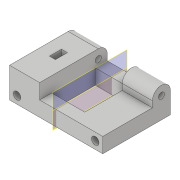
# Autodesk Inventor part: Carriage
Saved by Autodesk Inventor 2019 (Build 230136000, 136)
## iProperties
Created: 2019-01-26
Part Number: Carriage
Material: Generic
Document SubType Name: Modeling
Designer: Jared
Density: 1 g/cm^3
Appearance: Default
Author: Jared
Autodesk Inventor part; units mm, degrees
ref_plane "YZ Plane" through (0, 0, 0) normal (1, 0, 0) x (0, 1, 0)
ref_plane "XZ Plane" through (0, 0, 0) normal (0, 1, 0) x (-1, 0, 0)
ref_plane "XY Plane" through (0, 0, 0) normal (0, 0, 1) x (1, 0, 0)
sketch "Sketch1" plane through (0, 0, 0) normal (0, 1, 0) x (-1, 0, 0)
  line L0 (0, 0) -> (0, -22.5)
  line L1 (0, -22.5) -> (31, -22.5)
  line L2 (31, -22.5) -> (31, 0)
  line L3 (31, 0) -> (0, 0)
  dimension "d0" = 22.5
  dimension "d1" = 31
  constraints: 8 end point, 3 perpendicular, 1 vertical
  measures "d0" distance of L0.start L0.end
  measures "d1" distance of L0.end L1.end
extrude "Extrusion1" add sketch "Sketch1" along normal blind 5
sketch "Sketch2" plane through (-31, 0, 0) normal (0, 0, 1) x (1, 0, 0)
  line L0 (0, 0) -> (31, 0) projected
  line L1 (31, 0) -> (31, 5) projected
  line L2 (0, 5) -> (31, 5) projected
  line L3 (0, 0) -> (0, 5) projected
  line L4 (0, 0) -> (0, 5) projected
  line L5 (0, 2.5) -> (2.5, 2.5)
  circle A0 centre (2.5, 2.5) radius 1.25
  dimension "d4" = 2.5
  dimension "d5" = 2.5
  constraints: 2 end point, 1 centre point, 1 coincident, 1 horizontal, 1 midpoint
  measures "d4" distance of L5.start L5.end
  measures "d5" diameter of A0
extrude "Extrusion2" cut sketch "Sketch2" against normal up to next contours A0
ref_plane "Work Plane1" through (-15.5, 0, 0) normal (1, 0, 0) x (0, 0, -1)
mirror "Mirror1" about plane through (-15.5, 0, 0) normal (1, 0, 0) of "Extrusion2"
sketch "Sketch3" plane through (0, 5, 0) normal (0, 1, 0) x (1, 0, 0)
  line L0 (0, 0) -> (0, 22.5) projected
  line L1 (0, 22.5) -> (-31, 22.5) projected
  line L2 (-31, 22.5) -> (-31, 0) projected
  line L3 (-31, 0) -> (0, 0) projected
  line L4 (0, 22.5) -> (-31, 22.5) projected
  line L5 (-15.5, 22.5) -> (-15.5, 18.5)
  line L6 (-31, 0) -> (0, 0) projected
  line L7 (-15.5, 0) -> (-15.5, 4)
  line L8 (-21, 18.5) -> (-10, 18.5)
  line L9 (-10, 18.5) -> (-10, 4)
  line L10 (-21, 4) -> (-21, 18.5)
  line L11 (-31, 22.5) -> (-31, 0) projected
  line L12 (-10, 4) -> (-15.5, 4)
  line L13 (-15.5, 4) -> (-21, 4)
  dimension "d8" = 4
  dimension "d9" = 4
  dimension "d11" = 11
  constraints: 14 end point, 3 midpoint, 2 equal length, 2 horizontal, 2 vertical, 1 collinear, 1 perpendicular
  measures "d8" distance of L5.start L5.end
  measures "d9" distance of L7.start L7.end
  measures "d11" distance of L8.start L8.end
extrude "Extrusion3" cut sketch "Sketch3" against normal up to next contours L13 L10 L8 L9 L12
sketch "Sketch4" plane through (0, 0, 0) normal (1, 0, 0) x (0, 0, -1)
  line L0 (0, 0) -> (22.5, 0) projected
  line L1 (22.5, 0) -> (22.5, 5) projected
  line L2 (0, 5) -> (22.5, 5) projected
  line L3 (0, 0) -> (0, 5) projected
  line L4 (0, 5) -> (22.5, 5) projected
  line L5 (22.5, 0) -> (22.5, 5) projected
  line L6 (22.5, 5) -> (22.5, 7)
  line L7 (22.5, 7) -> (19.5, 7)
  arc A0 (22.5, 7) -> (16.5, 7) centre (19.5, 7) ccw
  line L8 (16.5, 7) -> (16.5, 5)
  circle A1 centre (19.5, 7) radius 1
  dimension "d21" = 2
  dimension "d22" = 3
  dimension "d23" = 2
  constraints: 6 end point, 2 centre point, 2 coincident, 2 perpendicular, 2 point on circle, 2 point on line, 1 vertical
  measures "d21" distance of L1.end L6.end
  measures "d22" distance of L6.end L7.end
  measures "d23" diameter of A1
extrude "Extrusion4" add sketch "Sketch4" against normal blind 10 contours L2 L8 A0 L6
ref_plane "Work Plane2" through (-15.5, 0, -22.5) normal (-1, 0, 0) x (0, 0, 1)
mirror "Mirror2" about plane through (-15.5, 0, -22.5) normal (-1, 0, 0) of "Extrusion4"
sketch "Sketch6" plane through (-31, 0, -22.5) normal (-1, 0, 0) x (0, 0, 1)
  circle A0 centre (3, 7) radius 1 projected
  line L0 (0, 0) -> (22.5, 0) projected
  line L1 (22.5, 0) -> (22.5, 5) projected
  line L2 (6, 5) -> (22.5, 5) projected
  line L3 (6, 7) -> (6, 5) projected
  arc A1 (6, 7) -> (0, 7) centre (3, 7) ccw projected
  line L4 (0, 0) -> (0, 7) projected
  arc A2 (6, 7) -> (0, 7) centre (3, 7) ccw projected
  line L5 (3, 10) -> (22.5, 10)
  line L6 (6, 5) -> (22.5, 5) projected
  line L7 (22.5, 5) -> (22.5, 10)
  constraints: 4 end point, 2 point on circle, 1 horizontal, 1 perpendicular
extrude "Extrusion6" add sketch "Sketch6" against normal up to surface (10 mm away) contours L2 L3 A1 L5 L7
sketch "Sketch7" plane through (-31, 10, 0) normal (0, 1, 0) x (1, 0, 0)
  line L0 (10, 19.5) -> (10, 0) projected
  line L1 (10, 19.5) -> (0, 19.5) projected
  line L2 (0, 0) -> (0, 19.5) projected
  line L3 (0, 0) -> (10, 0) projected
  line L4 (6, 13.25) -> (4, 13.25)
  line L5 (4, 13.25) -> (4, 9.25)
  line L6 (4, 9.25) -> (6, 9.25)
  line L7 (6, 9.25) -> (6, 13.25)
  line L8 (0, 0) -> (0, 19.5) projected
  line L9 (0, 11.25) -> (4, 11.25)
  line L10 (6, 11.25) -> (10, 11.25)
  line L11 (10, 19.5) -> (10, 0) projected
  line L12 (0, 22.5) -> (10, 22.5) projected
  line L13 (5, 22.5) -> (5, 13.25)
  line L14 (5, 9.25) -> (5, 0)
  point P0 (31, 0)
  dimension "d28" = 2
  dimension "d29" = 4
  constraints: 16 end point, 6 midpoint, 3 perpendicular, 3 point on line, 2 collinear, 2 parallel, 1 horizontal
  measures "d28" distance of L5.end L6.end
  measures "d29" distance of L4.end L5.end
extrude "Extrusion7" cut sketch "Sketch7" against normal blind 5 contours L7 L6 L5 L4
body "Solid1"
